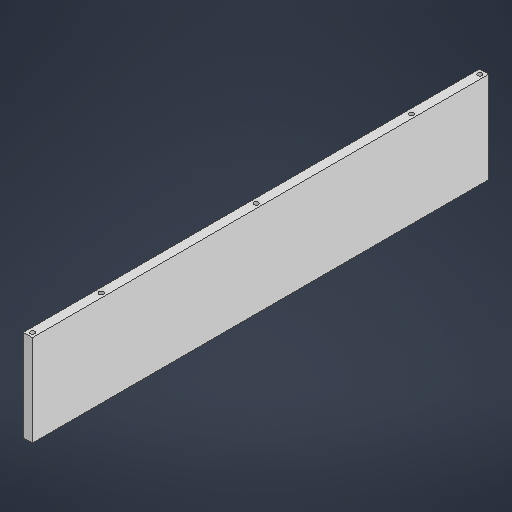
# Autodesk Inventor part: DindingRobotDepanBelakang
Saved by Autodesk Inventor 2026.1 (Build 301233020, 233B)
## iProperties
Created: 2025-11-08
Part Number: DindingRobotDepanBelakang
Material: Generic
Document SubType Name: Modeling
Designer: FrianVex
Density: 1 g/cm^3
Appearance: Default
Author: FrianVex
Autodesk Inventor part; units mm, degrees
ref_plane "YZ Plane" through (0, 0, 0) normal (1, 0, 0) x (0, 1, 0)
ref_plane "XZ Plane" through (0, 0, 0) normal (0, 1, 0) x (-1, 0, 0)
ref_plane "XY Plane" through (0, 0, 0) normal (0, 0, 1) x (1, 0, 0)
sketch "Sketch1" plane through (0, 0, 0) normal (0, 1, 0) x (-1, 0, 0)
  line L0 (-2, -100) -> (2, -100)
  line L1 (2, -100) -> (2, 100)
  line L2 (2, 100) -> (-2, 100)
  line L3 (-2, 100) -> (-2, -100)
  line L4 (-2, -100) -> (2, 100) construction
  line L5 (2, -100) -> (-2, 100) construction
  circle A0 centre (-0.1, 98) radius 1
  circle A1 centre (-0.1, 68) radius 1
  circle A2 centre (-0.1, 0) radius 1
  circle A3 centre (-0.1, -98) radius 1
  circle A4 centre (-0.1, -68) radius 1
  point P0 (0, 0)
  dimension "d0" = 4
  dimension "d1" = 200
  dimension "d2" = 2
  dimension "d3" = 2.1
  dimension "d4" = 2
  dimension "d5" = 2
  dimension "d6" = 32
  dimension "d7" = 2.1
  dimension "d8" = 2
  dimension "d9" = 100
  dimension "d10" = 2.1
  dimension "d11" = 2
  dimension "d12" = 2
  dimension "d13" = 2.1
  dimension "d14" = 2
  dimension "d15" = 2.1
  dimension "d16" = 32
  constraints: 12 end point, 5 centre point, 2 midpoint, 2 parallel, 1 horizontal, 1 perpendicular
  measures "d0" distance of L2.end L1.end
  measures "d1" distance of L0.end L1.end
  measures "d2" diameter of A0
  measures "d3" distance from line of L1 A0.centre
  measures "d4" distance from line of L2 A0.centre
  measures "d5" diameter of A1
  measures "d6" distance from line of L2 A1.centre
  measures "d7" distance from line of L1 A1.centre
  measures "d8" diameter of A2
  measures "d9" distance from line of L2 A2.centre
  measures "d10" distance from line of L1 A2.centre
  measures "d11" diameter of A3
  measures "d12" distance from line of L0 A3.centre
  measures "d13" distance from line of L1 A3.centre
  measures "d14" diameter of A4
  measures "d15" distance from line of L1 A4.centre
  measures "d16" distance from line of L0 A4.centre
extrude "Extrusion1" add sketch "Sketch1" along normal blind 40
body "Solid1"
